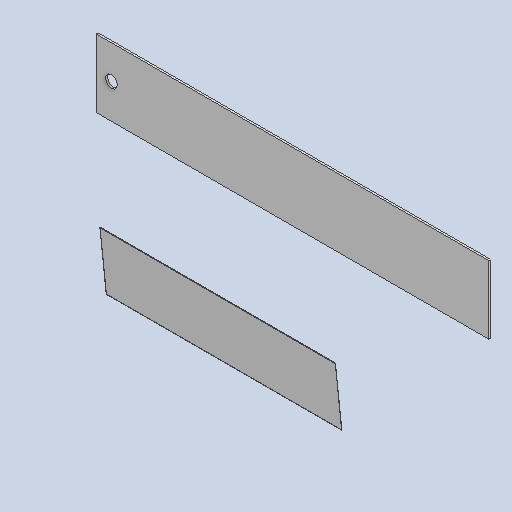
# Autodesk Inventor part: pokrywa tylna
Saved by Autodesk Inventor 2023 (Build 270158000, 158)
## iProperties
Created: 2023-08-18
Part Number: pokrywa tylna
Material: Ogólny
Document SubType Name: Modeling
Designer: Kamil
Density: 1 g/cm^3
Appearance: Domyślna
Author: Kamil
Autodesk Inventor part; units mm, degrees
ref_plane "YZ Plane" through (0, 0, 0) normal (1, 0, 0) x (0, 1, 0)
ref_plane "XZ Plane" through (0, 0, 0) normal (0, 1, 0) x (-1, 0, 0)
ref_plane "XY Plane" through (0, 0, 0) normal (0, 0, 1) x (1, 0, 0)
sketch "Szkic1" plane through (0, 0, 0) normal (0, 0, 1) x (1, 0, 0)
  line L0 (-0.6, 0) -> (-0.6, 13.1255)
  line L1 (2.7848, 0) -> (-0.6, 0)
  spline S0 degree 3 poles (3.0833, 0.1968) (3.0705, 0.1915) (3.0579, 0.186) (2.9555, 0.1384) (2.8611, 0.0732) (2.7848, 0) knots 0 0 0 0 0.118922 0.118922 1 1 1 1
  spline S1 degree 3 poles (3.0833, 0.1968) (3.1541, 0.2257) (3.223, 0.256) (3.5835, 0.4251) (3.888, 0.6087) (4.4504, 1.0382) (4.7087, 1.2836) (5.1613, 1.7912) (5.3932, 2.1042) (5.7913, 2.77) (5.9577, 3.1227) (6.2121, 3.7972) (6.3223, 4.1828) (6.4663, 4.968) (6.5, 5.3675) (6.5, 5.7331) knots -1.428143 -1.428143 -1.428143 -1.428143 -1.406087 -1.406087 -1.308684 -1.308684 -1.211282 -1.211282 -1.104676 -1.104676 -0.99807 -0.99807 -0.888411 -0.888411 -0.778752 -0.778752 -0.778752 -0.778752
  line L2 (6.5, 5.7331) -> (6.5, 13.1255)
  line L3 (6.5, 13.1255) -> (-0.6, 13.1255)
  circle A0 centre (3.25, 5.9055) radius 1.5
  line L4 (99.4, 0.1219) -> (99.4, 13.1642)
  line L5 (92.3, 13.1642) -> (99.4, 13.1642)
  line L6 (92.3, 0.1219) -> (92.3, 13.1642)
  line L7 (92.3, 0.1219) -> (99.4, 0.1219)
  line L8 (-0.6, 13.1255) -> (99.4, 13.1255)
  line L9 (99.4, 13.1255) -> (99.4, 0.1219)
  line L10 (99.4, 0.1219) -> (-0.6, 0.1219)
  line L11 (-0.6, 0.1219) -> (-0.6, 13.1255)
  line L12 (-0.6, 0.1219) -> (99.4, 0.1219)
  line L13 (99.4, 0.1219) -> (99.4, -2.8781)
  line L14 (99.4, -2.8781) -> (-0.6, -2.8781)
  line L15 (-0.6, -2.8781) -> (-0.6, 0.1219)
  line L16 (19.4, 0.1219) -> (79.4, 0.1219)
  line L17 (79.4, 0.1219) -> (79.4, -19.8781)
  line L18 (79.4, -19.8781) -> (19.4, -19.8781)
  line L19 (19.4, -19.8781) -> (19.4, 0.1219)
  ellipse E0 centre (2.95, 26.8204) end of major axis (4.45, 26.8204) minor radius 0.3241
  ellipse E1 centre (49.4, 17.3721) end of major axis (50.4, 17.3721) minor radius 0.2161
  ellipse E2 centre (73.9, 17.3721) end of major axis (74.9, 17.3721) minor radius 0.2161
  ellipse E3 centre (24.9, 19.4245) end of major axis (25.9, 19.4245) minor radius 0.2161
  ellipse E4 centre (95.85, 26.8204) end of major axis (97.35, 26.8204) minor radius 0.3241
  ellipse E5 centre (2.95, 16.7506) end of major axis (4.45, 16.7506) minor radius 0.3241
  ellipse E6 centre (49.4, 19.4245) end of major axis (50.4, 19.4245) minor radius 0.2161
  ellipse E7 centre (73.9, 19.4245) end of major axis (74.9, 19.4245) minor radius 0.2161
  ellipse E8 centre (24.9, 17.3721) end of major axis (25.9, 17.3721) minor radius 0.2161
  ellipse E9 centre (95.85, 16.7506) end of major axis (97.35, 16.7506) minor radius 0.3241
  ellipse E10 centre (44.2014, 21.2376) end of major axis (46.7514, 21.2376) minor radius 0.5509
  ellipse E11 centre (35.3114, 21.2376) end of major axis (37.8614, 21.2376) minor radius 0.5509
  ellipse E12 centre (53.0914, 21.2376) end of major axis (55.6414, 21.2376) minor radius 0.5509
  line L20 (28.3783, 20.6632) -> (17.5183, 20.6632)
  line L21 (17.5183, 20.6632) -> (17.5183, 21.3633)
  line L22 (17.5183, 21.3633) -> (28.3783, 21.3633)
  line L23 (28.3783, 21.3633) -> (28.3783, 20.6632)
  line L24 (77.2802, 20.6127) -> (77.2802, 22.1251)
  line L25 (77.2802, 22.1251) -> (84.2802, 22.1251)
  line L26 (84.2802, 22.1251) -> (84.2802, 20.6127)
  line L27 (84.2802, 20.6127) -> (77.2802, 20.6127)
  line L28 (99.4, 14.3474) -> (99.4, 29.4709)
  line L29 (99.4, 29.4709) -> (-0.6, 29.4709)
  line L30 (-0.6, 29.4709) -> (-0.6, 14.3474)
  line L31 (-0.6, 14.3474) -> (99.4, 14.3474)
  line L32 (99.4, 13.1255) -> (-0.6, 13.1255)
  line L33 (-0.6, 13.1255) -> (-0.6, 14.3474)
  line L34 (-0.6, 14.3474) -> (99.4, 14.3474)
  line L35 (99.4, 14.3474) -> (99.4, 13.1255)
  ellipse E13 centre (95.55, 5.99) end of major axis (97.05, 5.99) minor radius 1.4905
  point P0 (0, 0)
  point P1 (49.4, 0.1219)
  point P2 (49.4, 0.1219)
  point P3 (49.4, 0.1219)
  point P4 (19.4, -2.8781)
  point P5 (79.4, -2.8781)
  point P6 (92.3, 13.1255)
  point P7 (2.9401, 0.1219)
  point P8 (92.3, 13.1255)
  dimension "d0" = 3
  dimension "d1" = 60
  dimension "d2" = 20
  constraints: 32 end point, 8 parallel, 4 horizontal, 4 perpendicular, 3 midpoint, 2 coincident
  measures "d0" distance of L12.end L13.end
  measures "d1" distance of L17.end L18.end
  measures "d2" distance of L16.end L17.end
extrude "Wyciągnięcie proste1" add sketch "Szkic1" along normal blind 0.5 contours L0 L10 S0 L1 | L1 S0 L10 L19 L14 L15 | L0 L3 L2 S1 S0 L10 | S0 S1 L2 L8 L6 L10 | L19 L10 L17 L14 | L14 L17 L18 L19 | L17 L10 L7 L13 L14 | L8 L4 L7 L6 | E13
sketch "Szkic2" plane through (-0.6, -2.8781, 0) normal (-1, 0, 0) x (0, 0, 1)
  line L0 (0, 16.0036) -> (0, 0) projected
  line L1 (0, 0) -> (0.5, 0) projected
  line L2 (0.5, 16.0036) -> (0.5, 0) projected
  line L3 (0, 16.0036) -> (0.5, 16.0036) projected
  line L4 (0.5, 16.0036) -> (0, 16.0036)
  line L5 (0, 16.0036) -> (0, 17.3406)
  line L6 (0, 17.3406) -> (0.5, 17.3406)
  line L7 (0.5, 17.3406) -> (0.5, 16.0036)
  point P0 (0, 2.8781)
  constraints: 8 end point, 2 parallel, 1 horizontal, 1 perpendicular
ref_plane "Płaszczyzna konstrukcyjna1" through (99.4, 13.8592, -68.0339) normal (1, 0, 0) x (0, 0.9763823, 0.2160502)
extrude "Wyciągnięcie proste2" add sketch "Szkic2" against normal up to surface (100 mm away) contours L5 L6 L7 L3
sketch "Szkic3" plane through (19.4, -19.8781, 0) normal (-1, 0, 0) x (0, 0, 1)
  line L0 (0, 17) -> (0, 0) projected
  line L1 (0, 0) -> (0.5, 0) projected
  line L2 (0.5, 17) -> (0.5, 0) projected
  line L3 (0, 17) -> (0.5, 17) projected
  line L4 (18.2345, -1.363) -> (19.5458, 11.068) projected
  line L5 (17.9197, -4.3465) -> (18.2345, -1.363) projected
  line L6 (17.9197, -4.3465) -> (18.417, -4.3989)
  line L7 (18.417, -4.3989) -> (0.5, -174.2432)
  line L8 (19.5458, 11.068) -> (19.6488, 11.5332)
  line L9 (0.5, -174.2432) -> (19.6018, 11.3211)
  point P0 (0, 19.8781)
  point P1 (0.0183, 10.8546)
  point P2 (17.9883, -4.3537)
  dimension "d7" = 0.5
  constraints: 8 end point, 2 perpendicular, 2 point on line
  measures "d7" distance of L5.start L6.end
extrude "Wyciągnięcie proste3" add sketch "Szkic3" against normal up to surface (60 mm away) contours L4 L8 L9 L6 L5
sketch "Szkic4" plane through (19.4, -19.8781, 0.5) normal (-1, 0, 0) x (0, 0, 1)
  line L0 (-0.5, 17) -> (-0.5, 0) projected
  line L1 (-0.5, 0) -> (0, 0) projected
  line L2 (0, 17) -> (0, 0) projected
  line L3 (-0.5, 17) -> (0, 17) projected
  line L4 (-0.5, 0) -> (-0.5, 17) projected
  line L5 (-0.5, 8.7524) -> (0.9116, 15.1318)
  point P0 (-0.5, 19.8781)
  point P1 (0, 11.012)
  constraints: 2 end point
extrude "Wyciągnięcie proste4" cut sketch "Szkic4" against normal through all
sketch "Szkic5" plane through (19.4, -24.3493, -2.8991) normal (0, -0.2160502, 0.9763823) x (1, 0, 0)
  ellipse E0 centre (55, 12.4499) end of major axis (56, 12.4499) minor radius 0.9937 projected
  ellipse E1 centre (5, 12.4499) end of major axis (6, 12.4499) minor radius 0.9937 projected
  point P0 (-19.4, 24.4006)
extrude "Wyciągnięcie proste5" [suppressed]
